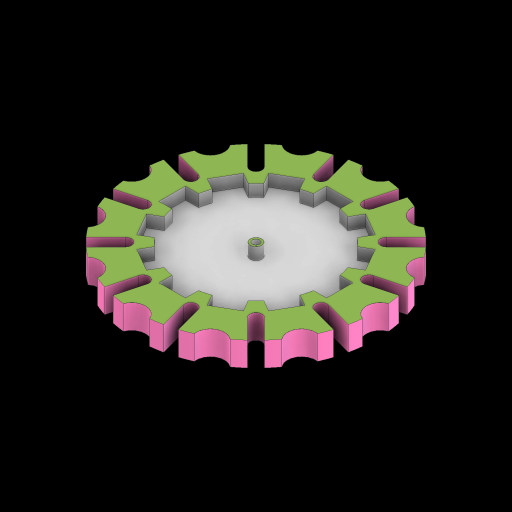
# Autodesk Inventor part: SC-1-02-Geneva Gear 12
Saved by Autodesk Inventor 2023 (Build 270158000, 158)
## iProperties
Created: 2022-10-22
Part Number: SC-1-02-Geneva Gear 12
Material: Generic
Document SubType Name: Modeling
Designer: annah
Density: 1 g/cm^3
Appearance: Default
Author: annah
Autodesk Inventor part; units mm, degrees
ref_plane "YZ Plane" through (0, 0, 0) normal (1, 0, 0) x (0, 1, 0)
ref_plane "XZ Plane" through (0, 0, 0) normal (0, 1, 0) x (-1, 0, 0)
ref_plane "XY Plane" through (0, 0, 0) normal (0, 0, 1) x (1, 0, 0)
sketch "Sketch1" plane through (0, 0, 0) normal (0, 1, 0) x (-1, 0, 0)
  line L0 (19.1342, -46.194) -> (0, -54.1231)
  line L1 (0, -54.1231) -> (0, 0)
  line L2 (0, 0) -> (19.1342, -46.194)
  circle A0 centre (0, 0) radius 50
  line L3 (17.2491, -28.6141) -> (23.8838, -44.6316)
  circle A1 centre (0, -54.1231) radius 20.712
  arc A2 (17.5355, -29.3054) -> (8.1665, -32.7812) centre (12.7859, -30.8678) ccw
  line L4 (14.5151, -48.1081) -> (8.1665, -32.7812)
  line L5 (19.1342, -41.194) -> (0, -41.194)
  circle A3 centre (0, -54.1231) radius 12.9291
  arc A4 (-11.6961, -48.6128) -> (11.6961, -48.6128) centre (0, 0) ccw
  arc A5 (-11.6961, -48.6128) -> (11.6961, -48.6128) centre (0, -54.1231) ccw
  circle A6 centre (0, -54.1231) radius 32.5
  arc A7 (19.1342, -41.194) -> (16.6765, -41.8397) centre (19.1342, -46.194) ccw
  arc A8 (14.4249, -47.874) -> (23.5974, -43.9403) centre (19.1342, -46.194) ccw
  line L6 (32.4302, -8.0362) -> (48.4477, -14.6709)
  arc A9 (33.1215, -8.3226) -> (28.9544, -17.4053) centre (30.8678, -12.7859) ccw
  line L7 (44.2813, -23.7539) -> (28.9544, -17.4053)
  arc A10 (44.052, -23.6521) -> (47.7564, -14.3846) centre (46.194, -19.1342) ccw
  circle A11 centre (38.2708, -38.2708) radius 12.9291
  line L8 (28.6141, 17.2491) -> (44.6316, 23.8838)
  arc A12 (29.3054, 17.5355) -> (32.7812, 8.1665) centre (30.8678, 12.7859) ccw
  line L9 (48.1081, 14.5151) -> (32.7812, 8.1665)
  arc A13 (47.874, 14.4249) -> (43.9403, 23.5974) centre (46.194, 19.1342) ccw
  circle A14 centre (54.1231, 0) radius 12.9291
  line L10 (8.0362, 32.4302) -> (14.6709, 48.4477)
  arc A15 (8.3226, 33.1215) -> (17.4053, 28.9544) centre (12.7859, 30.8678) ccw
  line L11 (23.7539, 44.2813) -> (17.4053, 28.9544)
  arc A16 (23.6521, 44.052) -> (14.3846, 47.7564) centre (19.1342, 46.194) ccw
  circle A17 centre (38.2708, 38.2708) radius 12.9291
  line L12 (-17.2491, 28.6141) -> (-23.8838, 44.6316)
  arc A18 (-17.5355, 29.3054) -> (-8.1665, 32.7812) centre (-12.7859, 30.8678) ccw
  line L13 (-14.5151, 48.1081) -> (-8.1665, 32.7812)
  arc A19 (-14.4249, 47.874) -> (-23.5974, 43.9403) centre (-19.1342, 46.194) ccw
  circle A20 centre (0, 54.1231) radius 12.9291
  line L14 (-32.4302, 8.0362) -> (-48.4477, 14.6709)
  arc A21 (-33.1215, 8.3226) -> (-28.9544, 17.4053) centre (-30.8678, 12.7859) ccw
  line L15 (-44.2813, 23.7539) -> (-28.9544, 17.4053)
  arc A22 (-44.052, 23.6521) -> (-47.7564, 14.3846) centre (-46.194, 19.1342) ccw
  circle A23 centre (-38.2708, 38.2708) radius 12.9291
  line L16 (-28.6141, -17.2491) -> (-44.6316, -23.8838)
  arc A24 (-29.3054, -17.5355) -> (-32.7812, -8.1665) centre (-30.8678, -12.7859) ccw
  line L17 (-48.1081, -14.5151) -> (-32.7812, -8.1665)
  arc A25 (-47.874, -14.4249) -> (-43.9403, -23.5974) centre (-46.194, -19.1342) ccw
  circle A26 centre (-54.1231, 0) radius 12.9291
  line L18 (-8.0362, -32.4302) -> (-14.6709, -48.4477)
  arc A27 (-8.3226, -33.1215) -> (-17.4053, -28.9544) centre (-12.7859, -30.8678) ccw
  line L19 (-23.7539, -44.2813) -> (-17.4053, -28.9544)
  arc A28 (-23.6521, -44.052) -> (-14.3846, -47.7564) centre (-19.1342, -46.194) ccw
  circle A29 centre (-38.2708, -38.2708) radius 12.9291
  circle A30 centre (0, 0) radius 3.5
  circle A31 centre (0, -54.1231) radius 3.5
  arc A32 (-7.5, -54.1231) -> (7.5, -54.1231) centre (0, -54.1231) ccw
  arc A33 (7.5, 0) -> (-7.5, 0) centre (0, 0) ccw
  line L20 (7.5, 0) -> (7.5, -54.1231)
  line L21 (-7.5, 0) -> (-7.5, -54.1231)
  circle A34 centre (0, -33.4111) radius 5
  point P0 (8.1662, -32.7805)
  point P1 (23.5974, -43.9403)
  point P2 (28.9537, -17.405)
  point P3 (29.1285, -29.1285)
  point P4 (26.1041, -42.6448)
  point P5 (42.6448, -26.1041)
  point P6 (32.7805, 8.1662)
  point P7 (41.194, 0)
  point P8 (48.6128, -11.6961)
  point P9 (48.6128, 11.6961)
  point P10 (17.405, 28.9537)
  point P11 (29.1285, 29.1285)
  point P12 (42.6448, 26.1041)
  point P13 (26.1041, 42.6448)
  point P14 (-8.1662, 32.7805)
  point P15 (0, 41.194)
  point P16 (11.6961, 48.6128)
  point P17 (-11.6961, 48.6128)
  point P18 (-28.9537, 17.405)
  point P19 (-29.1285, 29.1285)
  point P20 (-26.1041, 42.6448)
  point P21 (-42.6448, 26.1041)
  point P22 (-32.7805, -8.1662)
  point P23 (-41.194, 0)
  point P24 (-48.6128, 11.6961)
  point P25 (-48.6128, -11.6961)
  point P26 (-17.405, -28.9537)
  point P27 (-29.1285, -29.1285)
  point P28 (-42.6448, -26.1041)
  point P29 (-26.1041, -42.6448)
  point P30 (23.6521, -44.052)
  point P31 (26.1041, -42.6448)
  point P32 (42.6448, -26.1041)
  point P33 (44.049, -23.6577)
  point P34 (47.874, -14.4249)
  point P35 (48.6128, -11.6961)
  point P36 (48.6128, 11.6961)
  point P37 (47.8758, 14.4189)
  point P38 (44.052, 23.6521)
  point P39 (42.6448, 26.1041)
  point P40 (26.1041, 42.6448)
  point P41 (23.6577, 44.049)
  point P42 (14.4249, 47.874)
  point P43 (11.6961, 48.6128)
  point P44 (-11.6961, 48.6128)
  point P45 (-14.4189, 47.8758)
  point P46 (-23.6521, 44.052)
  point P47 (-26.1041, 42.6448)
  point P48 (-42.6448, 26.1041)
  point P49 (-44.049, 23.6577)
  point P50 (-47.874, 14.4249)
  point P51 (-48.6128, 11.6961)
  point P52 (-48.6128, -11.6961)
  point P53 (-47.8758, -14.4189)
  point P54 (-44.052, -23.6521)
  point P55 (-42.6448, -26.1041)
  point P56 (-26.1041, -42.6448)
  point P57 (-23.6577, -44.049)
  point P58 (-14.4249, -47.874)
  point P59 (14.4189, -47.8758)
  dimension "d2" = 100
  dimension "d3" = 22.5
  dimension "d4" = 20.712
  dimension "d5" = 50
  dimension "d6" = 54.1231
  dimension "d7" = 10
  dimension "d8" = 25.8582
  dimension "d9" = 65
  dimension "d10" = 360
  dimension "d11" = 7
  dimension "d12" = 7
  dimension "d13" = 15
  dimension "d14" = 15
  dimension "d15" = 10
  constraints: 113 point on circle, 44 end point, 35 centre point, 28 point on line, 9 coincident, 3 tangent, 2 vertical, 1 concentric, 1 parallel, 1 perpendicular, 161 other
  measures "d2" diameter of A0
  measures "d3" angle of L2 L1
  measures "d4" distance of L0.start L0.end
  measures "d5" distance of L1.end L0.start
  measures "d6" distance of L0.end L1.end
  measures "d7" diameter of A2
  measures "d8" diameter of A3
  measures "d9" diameter of A6
  measures "d11" diameter of A30
  measures "d12" diameter of A31
  measures "d13" diameter of A32
  measures "d14" diameter of A33
  measures "d15" diameter of A34
sketch "Sketch2" plane through (0, 0, 0) normal (0, 1, 0) x (-1, 0, 0)
  circle A0 centre (0, 0) radius 100
  line L0 (0, 0) -> (18.5658, -69.2885)
  line L1 (0, 0) -> (0, -103.5276)
  arc A1 (24.6448, -72.6673) -> (14.9907, -75.2542) centre (0, 0) ccw
  circle A2 centre (25.8819, -96.5926) radius 5
  arc A3 (24.729, -72.9816) -> (15.0747, -75.5678) centre (19.8599, -74.1181) ccw
  line L2 (30.6777, -95.1782) -> (24.6448, -72.6673)
  line L3 (21.0523, -97.8867) -> (14.9907, -75.2542)
  circle A4 centre (0, -103.5276) radius 11.6229
  line L4 (21.0523, -97.8867) -> (25.8819, -96.5926)
  arc A5 (-25.8819, -96.5926) -> (26.7197, -101.5219) centre (0, -103.5276) ccw
  circle A6 centre (0, -103.5276) radius 40
  arc A7 (57.9067, -50.8394) -> (50.8389, -57.9063) centre (54.2582, -54.2582) ccw
  line L5 (67.1751, -74.2462) -> (50.6094, -57.6767)
  line L6 (74.1567, -67.0879) -> (57.6767, -50.6094)
  circle A8 centre (70.7107, -70.7107) radius 5
  circle A9 centre (51.7638, -89.6575) radius 11.6229
  arc A10 (75.5684, -15.0748) -> (72.9809, -24.7289) centre (74.1181, -19.8599) ccw
  line L7 (95.2985, -30.7115) -> (72.6673, -24.6448)
  line L8 (97.7655, -21.0214) -> (75.2542, -14.9907)
  circle A11 centre (96.5926, -25.8819) radius 5
  circle A12 centre (89.6575, -51.7638) radius 11.6229
  arc A13 (72.9816, 24.729) -> (75.5678, 15.0747) centre (74.1181, 19.8599) ccw
  line L9 (97.8867, 21.0523) -> (75.2542, 14.9907)
  line L10 (95.1782, 30.6777) -> (72.6673, 24.6448)
  circle A14 centre (96.5926, 25.8819) radius 5
  circle A15 centre (103.5276, 0) radius 11.6229
  arc A16 (50.8394, 57.9067) -> (57.9063, 50.8389) centre (54.2582, 54.2582) ccw
  line L11 (74.2462, 67.1751) -> (57.6767, 50.6094)
  line L12 (67.0879, 74.1567) -> (50.6094, 57.6767)
  circle A17 centre (70.7107, 70.7107) radius 5
  circle A18 centre (89.6575, 51.7638) radius 11.6229
  arc A19 (15.0748, 75.5684) -> (24.7289, 72.9809) centre (19.8599, 74.1181) ccw
  line L13 (30.7115, 95.2985) -> (24.6448, 72.6673)
  line L14 (21.0214, 97.7655) -> (14.9907, 75.2542)
  circle A20 centre (25.8819, 96.5926) radius 5
  circle A21 centre (51.7638, 89.6575) radius 11.6229
  arc A22 (-24.729, 72.9816) -> (-15.0747, 75.5678) centre (-19.8599, 74.1181) ccw
  line L15 (-21.0523, 97.8867) -> (-14.9907, 75.2542)
  line L16 (-30.6777, 95.1782) -> (-24.6448, 72.6673)
  circle A23 centre (-25.8819, 96.5926) radius 5
  circle A24 centre (0, 103.5276) radius 11.6229
  arc A25 (-57.9067, 50.8394) -> (-50.8389, 57.9063) centre (-54.2582, 54.2582) ccw
  line L17 (-67.1751, 74.2462) -> (-50.6094, 57.6767)
  line L18 (-74.1567, 67.0879) -> (-57.6767, 50.6094)
  circle A26 centre (-70.7107, 70.7107) radius 5
  circle A27 centre (-51.7638, 89.6575) radius 11.6229
  arc A28 (-75.5684, 15.0748) -> (-72.9809, 24.7289) centre (-74.1181, 19.8599) ccw
  line L19 (-95.2985, 30.7115) -> (-72.6673, 24.6448)
  line L20 (-97.7655, 21.0214) -> (-75.2542, 14.9907)
  circle A29 centre (-96.5926, 25.8819) radius 5
  circle A30 centre (-89.6575, 51.7638) radius 11.6229
  arc A31 (-72.9816, -24.729) -> (-75.5678, -15.0747) centre (-74.1181, -19.8599) ccw
  line L21 (-97.8867, -21.0523) -> (-75.2542, -14.9907)
  line L22 (-95.1782, -30.6777) -> (-72.6673, -24.6448)
  circle A32 centre (-96.5926, -25.8819) radius 5
  circle A33 centre (-103.5276, 0) radius 11.6229
  arc A34 (-50.8394, -57.9067) -> (-57.9063, -50.8389) centre (-54.2582, -54.2582) ccw
  line L23 (-74.2462, -67.1751) -> (-57.6767, -50.6094)
  line L24 (-67.0879, -74.1567) -> (-50.6094, -57.6767)
  circle A35 centre (-70.7107, -70.7107) radius 5
  circle A36 centre (-89.6575, -51.7638) radius 11.6229
  arc A37 (-15.0748, -75.5684) -> (-24.7289, -72.9809) centre (-19.8599, -74.1181) ccw
  line L25 (-30.7115, -95.2985) -> (-24.6448, -72.6673)
  line L26 (-21.0214, -97.7655) -> (-14.9907, -75.2542)
  circle A38 centre (-25.8819, -96.5926) radius 5
  circle A39 centre (-51.7638, -89.6575) radius 11.6229
  circle A40 centre (0, 0) radius 3
  circle A41 centre (0, -103.5276) radius 2.5
  point P0 (50.7227, -50.7227)
  point P1 (73.9009, -74.5607)
  point P2 (69.2885, -18.5658)
  point P3 (101.2804, -27.621)
  point P4 (69.2885, 18.5658)
  point P5 (101.5219, 26.7197)
  point P6 (50.7227, 50.7227)
  point P7 (74.5607, 73.9009)
  point P8 (18.5658, 69.2885)
  point P9 (27.621, 101.2804)
  point P10 (-18.5658, 69.2885)
  point P11 (-26.7197, 101.5219)
  point P12 (-50.7227, 50.7227)
  point P13 (-73.9009, 74.5607)
  point P14 (-69.2885, 18.5658)
  point P15 (-101.2804, 27.621)
  point P16 (-69.2885, -18.5658)
  point P17 (-101.5219, -26.7197)
  point P18 (-50.7227, -50.7227)
  point P19 (-74.5607, -73.9009)
  point P20 (-18.5658, -69.2885)
  point P21 (-27.621, -101.2804)
  point P22 (40.2917, -91.5236)
  point P23 (59.1159, -80.6555)
  point P24 (67.0867, -74.1578)
  point P25 (80.6555, -59.1159)
  point P26 (91.5236, -40.2917)
  point P27 (95.1777, -30.6791)
  point P28 (99.4077, -10.8682)
  point P29 (99.4077, 10.8682)
  point P30 (97.7659, 21.0199)
  point P31 (91.5236, 40.2917)
  point P32 (80.6555, 59.1159)
  point P33 (74.1578, 67.0867)
  point P34 (59.1159, 80.6555)
  point P35 (40.2917, 91.5236)
  point P36 (30.6791, 95.1777)
  point P37 (10.8682, 99.4077)
  point P38 (-10.8682, 99.4077)
  point P39 (-21.0199, 97.7659)
  point P40 (-40.2917, 91.5236)
  point P41 (-59.1159, 80.6555)
  point P42 (-67.0867, 74.1578)
  point P43 (-80.6555, 59.1159)
  point P44 (-91.5236, 40.2917)
  point P45 (-95.1777, 30.6791)
  point P46 (-99.4077, 10.8682)
  point P47 (-99.4077, -10.8682)
  point P48 (-97.7659, -21.0199)
  point P49 (-91.5236, -40.2917)
  point P50 (-80.6555, -59.1159)
  point P51 (-74.1578, -67.0867)
  point P52 (-59.1159, -80.6555)
  point P53 (-40.2917, -91.5236)
  point P54 (-30.6791, -95.1777)
  point P55 (-10.8682, -99.4077)
  point P56 (10.8682, -99.4077)
  point P57 (21.0199, -97.7659)
  dimension "d16" = 200
  dimension "d17" = 15
  dimension "d20" = 10
  dimension "d21" = 10
  dimension "d22" = 80
  dimension "d25" = 360
  dimension "d27" = 6
  dimension "d28" = 5
  constraints: 100 point on circle, 54 end point, 41 centre point, 25 point on line, 8 coincident, 1 vertical, 198 other
  measures "d17" angle of L1 L0
  measures "d20" diameter of A2
  measures "d21" diameter of A3
  measures "d22" diameter of A6
  measures "d27" diameter of A40
  measures "d28" diameter of A41
extrude "Extrusion1" add sketch "Sketch2" along normal blind 20 contours L26 A37 A1 L1 A4 A0 | A0 A6 A1 A37 L25 | A0 A39 L24 A34 A1 A6 | L1 A1 A3 L3 A0 A4 | A37 A6 L1 A1 | A6 A37 A1 | A1 A34 A31 A28 A25 A22 A19 A16 A13 A10 A7 A6 A3 L0 A40 L1 A37 | L1 A6 L0 A3 A1 | A6 A1 A7 L5 A0 A9 | A0 L2 A3 A1 A6 | L1 A40 L0 A6 | A34 L23 A0 A36 L22 A31 A1 | A1 A3 A6 | A6 A3 L0 | A31 L21 A0 A33 L20 A28 A1 | A1 A10 L7 A0 A12 L6 A7 | A28 L19 A0 A30 L18 A25 A1 | A1 A13 L9 A0 A15 L8 A10 | A25 L17 A0 A27 L16 A22 A1 | A1 A16 L11 A0 A18 L10 A13 | A22 L15 A0 A24 L14 A19 A1 | A1 A19 L13 A0 A21 L12 A16 picked at (-24.7526, -72.3861)
sketch "Sketch3" plane through (0, 20, 0) normal (0, 1, 0) x (1, 0, 0)
  circle A0 centre (0, 0) radius 3 projected
  line L0 (-11.0031, 74.0969) -> (11.0031, 74.0969)
  line L1 (11.0031, 74.0969) -> (11.0031, 56.269)
  line L2 (11.0031, 56.269) -> (-11.0031, 56.269)
  line L3 (-11.0031, 56.269) -> (-11.0031, 74.0969)
  line L4 (11.0031, 74.0969) -> (0, 65.183) construction
  line L5 (-27.5195, 69.6713) -> (-18.6056, 54.232)
  line L6 (-18.6056, 54.232) -> (-37.6635, 43.2289)
  line L7 (-37.6635, 43.2289) -> (-46.5774, 58.6682)
  line L8 (-46.5774, 58.6682) -> (-27.5195, 69.6713)
  line L9 (-58.6682, 46.5774) -> (-43.2289, 37.6635)
  line L10 (-43.2289, 37.6635) -> (-54.232, 18.6056)
  line L11 (-54.232, 18.6056) -> (-69.6713, 27.5195)
  line L12 (-69.6713, 27.5195) -> (-58.6682, 46.5774)
  line L13 (-74.0969, 11.0031) -> (-56.269, 11.0031)
  line L14 (-56.269, 11.0031) -> (-56.269, -11.0031)
  line L15 (-56.269, -11.0031) -> (-74.0969, -11.0031)
  line L16 (-74.0969, -11.0031) -> (-74.0969, 11.0031)
  line L17 (-69.6713, -27.5195) -> (-54.232, -18.6056)
  line L18 (-54.232, -18.6056) -> (-43.2289, -37.6635)
  line L19 (-43.2289, -37.6635) -> (-58.6682, -46.5774)
  line L20 (-58.6682, -46.5774) -> (-69.6713, -27.5195)
  line L21 (-46.5774, -58.6682) -> (-37.6635, -43.2289)
  line L22 (-37.6635, -43.2289) -> (-18.6056, -54.232)
  line L23 (-18.6056, -54.232) -> (-27.5195, -69.6713)
  line L24 (-27.5195, -69.6713) -> (-46.5774, -58.6682)
  line L25 (-11.0031, -74.0969) -> (-11.0031, -56.269)
  line L26 (-11.0031, -56.269) -> (11.0031, -56.269)
  line L27 (11.0031, -56.269) -> (11.0031, -74.0969)
  line L28 (11.0031, -74.0969) -> (-11.0031, -74.0969)
  line L29 (27.5195, -69.6713) -> (18.6056, -54.232)
  line L30 (18.6056, -54.232) -> (37.6635, -43.2289)
  line L31 (37.6635, -43.2289) -> (46.5774, -58.6682)
  line L32 (46.5774, -58.6682) -> (27.5195, -69.6713)
  line L33 (58.6682, -46.5774) -> (43.2289, -37.6635)
  line L34 (43.2289, -37.6635) -> (54.232, -18.6056)
  line L35 (54.232, -18.6056) -> (69.6713, -27.5195)
  line L36 (69.6713, -27.5195) -> (58.6682, -46.5774)
  line L37 (74.0969, -11.0031) -> (56.269, -11.0031)
  line L38 (56.269, -11.0031) -> (56.269, 11.0031)
  line L39 (56.269, 11.0031) -> (74.0969, 11.0031)
  line L40 (74.0969, 11.0031) -> (74.0969, -11.0031)
  line L41 (69.6713, 27.5195) -> (54.232, 18.6056)
  line L42 (54.232, 18.6056) -> (43.2289, 37.6635)
  line L43 (43.2289, 37.6635) -> (58.6682, 46.5774)
  line L44 (58.6682, 46.5774) -> (69.6713, 27.5195)
  line L45 (46.5774, 58.6682) -> (37.6635, 43.2289)
  line L46 (37.6635, 43.2289) -> (18.6056, 54.232)
  line L47 (18.6056, 54.232) -> (27.5195, 69.6713)
  line L48 (27.5195, 69.6713) -> (46.5774, 58.6682)
  arc A1 (-11.0031, 60.9667) -> (-20.9544, 58.3003) centre (0, 0) ccw
  arc A2 (20.9544, 58.3003) -> (11.0031, 60.9667) centre (0, 0) ccw
  arc A3 (47.2972, 40.0123) -> (40.0123, 47.2972) centre (0, 0) ccw
  arc A4 (-40.0123, 47.2972) -> (-47.2972, 40.0123) centre (0, 0) ccw
  arc A5 (-58.3003, 20.9544) -> (-60.9667, 11.0031) centre (0, 0) ccw
  arc A6 (-60.9667, -11.0031) -> (-58.3003, -20.9544) centre (0, 0) ccw
  arc A7 (-47.2972, -40.0123) -> (-40.0123, -47.2972) centre (0, 0) ccw
  arc A8 (-20.9544, -58.3003) -> (-11.0031, -60.9667) centre (0, 0) ccw
  arc A9 (11.0031, -60.9667) -> (20.9544, -58.3003) centre (0, 0) ccw
  arc A10 (40.0123, -47.2972) -> (47.2972, -40.0123) centre (0, 0) ccw
  arc A11 (58.3003, -20.9544) -> (60.9667, -11.0031) centre (0, 0) ccw
  arc A12 (60.9667, 11.0031) -> (58.3003, 20.9544) centre (0, 0) ccw
  dimension "d36" = 360
  constraints: 98 end point, 24 point on circle, 24 point on line, 12 centre point, 3 coincident, 2 parallel, 1 horizontal, 1 perpendicular, 97 other
sketch "Sketch4" plane through (0, 20, 0) normal (0, 1, 0) x (1, 0, 0)
  line L0 (11.5029, -60.4669) -> (-11.5031, -60.4669)
  line L1 (-11.5031, -60.4669) -> (-11.5031, -74.5969)
  line L2 (-11.5031, -74.5969) -> (11.5029, -74.5969)
  line L3 (11.5029, -60.4669) -> (11.5029, -74.5969)
  line L4 (40.1952, -46.6144) -> (20.2715, -58.1174)
  line L5 (40.1952, -46.6144) -> (47.2602, -58.8513)
  line L6 (27.3365, -70.3543) -> (47.2602, -58.8513)
  line L7 (20.2715, -58.1174) -> (27.3365, -70.3543)
  line L8 (58.1173, -20.2716) -> (46.6143, -40.1954)
  line L9 (58.1173, -20.2716) -> (70.3542, -27.3366)
  line L10 (58.8512, -47.2604) -> (70.3542, -27.3366)
  line L11 (46.6143, -40.1954) -> (58.8512, -47.2604)
  line L12 (60.4669, 11.5029) -> (60.4669, -11.5031)
  line L13 (60.4669, 11.5029) -> (74.5969, 11.5029)
  line L14 (74.5969, -11.5031) -> (74.5969, 11.5029)
  line L15 (60.4669, -11.5031) -> (74.5969, -11.5031)
  line L16 (46.6144, 40.1952) -> (58.1174, 20.2715)
  line L17 (46.6144, 40.1952) -> (58.8513, 47.2602)
  line L18 (70.3543, 27.3365) -> (58.8513, 47.2602)
  line L19 (58.1174, 20.2715) -> (70.3543, 27.3365)
  line L20 (20.2716, 58.1173) -> (40.1954, 46.6143)
  line L21 (20.2716, 58.1173) -> (27.3366, 70.3542)
  line L22 (47.2604, 58.8512) -> (27.3366, 70.3542)
  line L23 (40.1954, 46.6143) -> (47.2604, 58.8512)
  line L24 (-11.5029, 60.4669) -> (11.5031, 60.4669)
  line L25 (-11.5029, 60.4669) -> (-11.5029, 74.5969)
  line L26 (11.5031, 74.5969) -> (-11.5029, 74.5969)
  line L27 (11.5031, 60.4669) -> (11.5031, 74.5969)
  line L28 (-40.1952, 46.6144) -> (-20.2715, 58.1174)
  line L29 (-40.1952, 46.6144) -> (-47.2602, 58.8513)
  line L30 (-27.3365, 70.3543) -> (-47.2602, 58.8513)
  line L31 (-20.2715, 58.1174) -> (-27.3365, 70.3543)
  line L32 (-58.1173, 20.2716) -> (-46.6143, 40.1954)
  line L33 (-58.1173, 20.2716) -> (-70.3542, 27.3366)
  line L34 (-58.8512, 47.2604) -> (-70.3542, 27.3366)
  line L35 (-46.6143, 40.1954) -> (-58.8512, 47.2604)
  line L36 (-60.4669, -11.5029) -> (-60.4669, 11.5031)
  line L37 (-60.4669, -11.5029) -> (-74.5969, -11.5029)
  line L38 (-74.5969, 11.5031) -> (-74.5969, -11.5029)
  line L39 (-60.4669, 11.5031) -> (-74.5969, 11.5031)
  line L40 (-46.6144, -40.1952) -> (-58.1174, -20.2715)
  line L41 (-46.6144, -40.1952) -> (-58.8513, -47.2602)
  line L42 (-70.3543, -27.3365) -> (-58.8513, -47.2602)
  line L43 (-58.1174, -20.2715) -> (-70.3543, -27.3365)
  line L44 (-20.2716, -58.1173) -> (-40.1954, -46.6143)
  line L45 (-20.2716, -58.1173) -> (-27.3366, -70.3542)
  line L46 (-47.2604, -58.8512) -> (-27.3366, -70.3542)
  line L47 (-40.1954, -46.6143) -> (-47.2604, -58.8512)
  circle A0 centre (0, 0) radius 5
  line L48 (-11.0031, 74.0969) -> (11.0031, 74.0969)
  line L49 (11.0031, 74.0969) -> (11.0031, 56.269)
  line L50 (11.0031, 56.269) -> (-11.0031, 56.269)
  line L51 (-11.0031, 56.269) -> (-11.0031, 74.0969)
  line L52 (11.0031, 74.0969) -> (0, 65.183) construction
  line L53 (-27.5195, 69.6713) -> (-18.6056, 54.232)
  line L54 (-18.6056, 54.232) -> (-37.6635, 43.2289)
  line L55 (-37.6635, 43.2289) -> (-46.5774, 58.6682)
  line L56 (-46.5774, 58.6682) -> (-27.5195, 69.6713)
  line L57 (-58.6682, 46.5774) -> (-43.2289, 37.6635)
  line L58 (-43.2289, 37.6635) -> (-54.232, 18.6056)
  line L59 (-54.232, 18.6056) -> (-69.6713, 27.5195)
  line L60 (-69.6713, 27.5195) -> (-58.6682, 46.5774)
  line L61 (-74.0969, 11.0031) -> (-56.269, 11.0031)
  line L62 (-56.269, 11.0031) -> (-56.269, -11.0031)
  line L63 (-56.269, -11.0031) -> (-74.0969, -11.0031)
  line L64 (-74.0969, -11.0031) -> (-74.0969, 11.0031)
  line L65 (-69.6713, -27.5195) -> (-54.232, -18.6056)
  line L66 (-54.232, -18.6056) -> (-43.2289, -37.6635)
  line L67 (-43.2289, -37.6635) -> (-58.6682, -46.5774)
  line L68 (-58.6682, -46.5774) -> (-69.6713, -27.5195)
  line L69 (-46.5774, -58.6682) -> (-37.6635, -43.2289)
  line L70 (-37.6635, -43.2289) -> (-18.6056, -54.232)
  line L71 (-18.6056, -54.232) -> (-27.5195, -69.6713)
  line L72 (-27.5195, -69.6713) -> (-46.5774, -58.6682)
  line L73 (-11.0031, -74.0969) -> (-11.0031, -56.269)
  line L74 (-11.0031, -56.269) -> (11.0031, -56.269)
  line L75 (11.0031, -56.269) -> (11.0031, -74.0969)
  line L76 (11.0031, -74.0969) -> (-11.0031, -74.0969)
  line L77 (27.5195, -69.6713) -> (18.6056, -54.232)
  line L78 (18.6056, -54.232) -> (37.6635, -43.2289)
  line L79 (37.6635, -43.2289) -> (46.5774, -58.6682)
  line L80 (46.5774, -58.6682) -> (27.5195, -69.6713)
  line L81 (58.6682, -46.5774) -> (43.2289, -37.6635)
  line L82 (43.2289, -37.6635) -> (54.232, -18.6056)
  line L83 (54.232, -18.6056) -> (69.6713, -27.5195)
  line L84 (69.6713, -27.5195) -> (58.6682, -46.5774)
  line L85 (74.0969, -11.0031) -> (56.269, -11.0031)
  line L86 (56.269, -11.0031) -> (56.269, 11.0031)
  line L87 (56.269, 11.0031) -> (74.0969, 11.0031)
  line L88 (74.0969, 11.0031) -> (74.0969, -11.0031)
  line L89 (69.6713, 27.5195) -> (54.232, 18.6056)
  line L90 (54.232, 18.6056) -> (43.2289, 37.6635)
  line L91 (43.2289, 37.6635) -> (58.6682, 46.5774)
  line L92 (58.6682, 46.5774) -> (69.6713, 27.5195)
  line L93 (46.5774, 58.6682) -> (37.6635, 43.2289)
  line L94 (37.6635, 43.2289) -> (18.6056, 54.232)
  line L95 (18.6056, 54.232) -> (27.5195, 69.6713)
  line L96 (27.5195, 69.6713) -> (46.5774, 58.6682)
  arc A1 (-11.0031, 60.9667) -> (-20.9544, 58.3003) centre (0, 0) ccw
  arc A2 (20.9544, 58.3003) -> (11.0031, 60.9667) centre (0, 0) ccw
  arc A3 (47.2972, 40.0123) -> (40.0123, 47.2972) centre (0, 0) ccw
  arc A4 (-40.0123, 47.2972) -> (-47.2972, 40.0123) centre (0, 0) ccw
  arc A5 (-58.3003, 20.9544) -> (-60.9667, 11.0031) centre (0, 0) ccw
  arc A6 (-60.9667, -11.0031) -> (-58.3003, -20.9544) centre (0, 0) ccw
  arc A7 (-47.2972, -40.0123) -> (-40.0123, -47.2972) centre (0, 0) ccw
  arc A8 (-20.9544, -58.3003) -> (-11.0031, -60.9667) centre (0, 0) ccw
  arc A9 (11.0031, -60.9667) -> (20.9544, -58.3003) centre (0, 0) ccw
  arc A10 (40.0123, -47.2972) -> (47.2972, -40.0123) centre (0, 0) ccw
  arc A11 (58.3003, -20.9544) -> (60.9667, -11.0031) centre (0, 0) ccw
  arc A12 (60.9667, 11.0031) -> (58.3003, 20.9544) centre (0, 0) ccw
  circle A13 centre (0, 0) radius 59.8407
  line L97 (-69.6713, -11.0031) -> (-49.8173, -11.0031)
  line L98 (-49.8173, -11.0031) -> (-49.8173, 11.0031)
  line L99 (-49.8173, 11.0031) -> (-69.6713, 11.0031)
  line L100 (-69.6713, 11.0031) -> (-69.6713, -11.0031)
  line L101 (-74.0969, 11.0031) -> (-56.269, 11.0031)
  line L102 (-65.8387, -25.3067) -> (-54.8356, -44.3646)
  line L103 (-48.6446, -15.3797) -> (-65.8387, -25.3067)
  line L104 (-37.6415, -34.4376) -> (-48.6446, -15.3797)
  line L105 (-54.8356, -44.3646) -> (-37.6415, -34.4376)
  line L106 (-69.6713, -27.5195) -> (-54.232, -18.6056)
  line L107 (-44.3646, -54.8356) -> (-25.3067, -65.8387)
  line L108 (-34.4376, -37.6415) -> (-44.3646, -54.8356)
  line L109 (-15.3797, -48.6446) -> (-34.4376, -37.6415)
  line L110 (-25.3067, -65.8387) -> (-15.3797, -48.6446)
  line L111 (-46.5774, -58.6682) -> (-37.6635, -43.2289)
  line L112 (-11.0031, -69.6713) -> (11.0031, -69.6713)
  line L113 (-11.0031, -49.8173) -> (-11.0031, -69.6713)
  line L114 (11.0031, -49.8173) -> (-11.0031, -49.8173)
  line L115 (11.0031, -69.6713) -> (11.0031, -49.8173)
  line L116 (-11.0031, -74.0969) -> (-11.0031, -56.269)
  line L117 (25.3067, -65.8387) -> (44.3646, -54.8356)
  line L118 (15.3797, -48.6446) -> (25.3067, -65.8387)
  line L119 (34.4376, -37.6415) -> (15.3797, -48.6446)
  line L120 (44.3646, -54.8356) -> (34.4376, -37.6415)
  line L121 (27.5195, -69.6713) -> (18.6056, -54.232)
  line L122 (54.8356, -44.3646) -> (65.8387, -25.3067)
  line L123 (37.6415, -34.4376) -> (54.8356, -44.3646)
  line L124 (48.6446, -15.3797) -> (37.6415, -34.4376)
  line L125 (65.8387, -25.3067) -> (48.6446, -15.3797)
  line L126 (58.6682, -46.5774) -> (43.2289, -37.6635)
  line L127 (69.6713, -11.0031) -> (69.6713, 11.0031)
  line L128 (49.8173, -11.0031) -> (69.6713, -11.0031)
  line L129 (49.8173, 11.0031) -> (49.8173, -11.0031)
  line L130 (69.6713, 11.0031) -> (49.8173, 11.0031)
  line L131 (74.0969, -11.0031) -> (56.269, -11.0031)
  line L132 (65.8387, 25.3067) -> (54.8356, 44.3646)
  line L133 (48.6446, 15.3797) -> (65.8387, 25.3067)
  line L134 (37.6415, 34.4376) -> (48.6446, 15.3797)
  line L135 (54.8356, 44.3646) -> (37.6415, 34.4376)
  line L136 (69.6713, 27.5195) -> (54.232, 18.6056)
  line L137 (44.3646, 54.8356) -> (25.3067, 65.8387)
  line L138 (34.4376, 37.6415) -> (44.3646, 54.8356)
  line L139 (15.3797, 48.6446) -> (34.4376, 37.6415)
  line L140 (25.3067, 65.8387) -> (15.3797, 48.6446)
  line L141 (46.5774, 58.6682) -> (37.6635, 43.2289)
  line L142 (11.0031, 69.6713) -> (-11.0031, 69.6713)
  line L143 (11.0031, 49.8173) -> (11.0031, 69.6713)
  line L144 (-11.0031, 49.8173) -> (11.0031, 49.8173)
  line L145 (-11.0031, 69.6713) -> (-11.0031, 49.8173)
  line L146 (11.0031, 74.0969) -> (11.0031, 56.269)
  line L147 (-25.3067, 65.8387) -> (-44.3646, 54.8356)
  line L148 (-15.3797, 48.6446) -> (-25.3067, 65.8387)
  line L149 (-34.4376, 37.6415) -> (-15.3797, 48.6446)
  line L150 (-44.3646, 54.8356) -> (-34.4376, 37.6415)
  line L151 (-27.5195, 69.6713) -> (-18.6056, 54.232)
  line L152 (-54.8356, 44.3646) -> (-65.8387, 25.3067)
  line L153 (-37.6415, 34.4376) -> (-54.8356, 44.3646)
  line L154 (-48.6446, 15.3797) -> (-37.6415, 34.4376)
  line L155 (-65.8387, 25.3067) -> (-48.6446, 15.3797)
  point P0 (-58.6905, -20.6023)
  point P1 (-47.1875, -40.5261)
  point P2 (-40.5263, -47.1874)
  point P3 (-20.6025, -58.6904)
  point P4 (-11.5031, -61.1286)
  point P5 (11.5029, -61.1286)
  point P6 (20.6023, -58.6905)
  point P7 (40.5261, -47.1875)
  point P8 (47.1874, -40.5263)
  point P9 (58.6904, -20.6025)
  point P10 (61.1286, -11.5031)
  point P11 (61.1286, 11.5029)
  point P12 (58.6905, 20.6023)
  point P13 (47.1875, 40.5261)
  point P14 (40.5263, 47.1874)
  point P15 (20.6025, 58.6904)
  point P16 (11.5031, 61.1286)
  point P17 (-11.5029, 61.1286)
  point P18 (-20.6023, 58.6905)
  point P19 (-40.5261, 47.1875)
  point P20 (-47.1874, 40.5263)
  point P21 (-58.6904, 20.6025)
  point P22 (-61.1286, 11.5031)
  point P23 (-61.1286, -11.5029)
  point P24 (-58.3003, -20.9544)
  point P25 (-11.0031, -60.9667)
  point P26 (20.9544, -58.3003)
  point P27 (47.2972, -40.0123)
  point P28 (60.9667, -11.0031)
  point P29 (58.3003, 20.9544)
  point P30 (40.0123, 47.2972)
  point P31 (11.0031, 60.9667)
  point P32 (-20.9544, 58.3003)
  point P33 (-45.4384, -38.9392)
  point P34 (-38.9392, -45.4384)
  point P35 (-19.8812, -56.4415)
  point P36 (-11.0031, -58.8204)
  point P37 (11.0031, -58.8204)
  point P38 (19.8812, -56.4415)
  point P39 (38.9392, -45.4384)
  point P40 (45.4384, -38.9392)
  point P41 (56.4415, -19.8812)
  point P42 (58.8204, -11.0031)
  point P43 (58.8204, 11.0031)
  point P44 (56.4415, 19.8812)
  point P45 (45.4384, 38.9392)
  point P46 (38.9392, 45.4384)
  point P47 (19.8812, 56.4415)
  point P48 (11.0031, 58.8204)
  point P49 (-11.0031, 58.8204)
  point P50 (-19.8812, 56.4415)
  point P51 (-38.9392, 45.4384)
  point P52 (-45.4384, 38.9392)
  point P53 (-56.4415, 19.8812)
  point P54 (-58.8204, 11.0031)
  point P55 (-58.8204, -11.0031)
  point P56 (-56.4415, -19.8812)
  dimension "d48" = 360
  dimension "d55" = 360
  dimension "d56" = 360
  constraints: 312 end point, 60 point on line, 24 point on circle, 13 centre point, 4 coincident, 4 parallel, 3 horizontal, 2 perpendicular, 1 vertical, 341 other
extrude "Extrusion4" cut sketch "Sketch4" against normal blind 10 contours L75 L112 L73 L0 | L0 L73 A13 L75 | A13 L73 L74 L75 | L75 L115 L114 L113 L73 A13 L71 L110 L109 L108 L69 L67 L105 L104 L103 L65 L63 L97 L98 L99 L61 L59 L155 L154 L153 L57 L55 L150 L149 L148 L53 L51 L145 L144 L143 L49 L95 L140 L139 L138 L93 L91 L135 L134 L133 L89 L87 L130 L129 L128 L85 L83 L125 L124 L123 L81 L79 L120 L119 L118 L77 | L74 L113 L114 L115 | A13 L79 L4 L77 | L77 L78 L79 A13 | L77 L4 L79 L117 | A13 L69 L70 L71 | L71 L44 L69 A13 | L118 L119 L120 L78 | L70 L108 L109 L110 | L71 L107 L69 L44 | A13 L83 L8 L81 | L81 L82 L83 A13 | A13 L65 L66 L67 | L67 L40 L65 A13 | L8 L83 L122 L81 | L123 L124 L125 L82 | L66 L103 L104 L105 | L67 L102 L65 L40 | A13 L87 L12 L85 | L85 L86 L87 A13 | A13 L61 L62 L63 | L63 L36 L61 A13 | L12 L87 L127 L85 | L128 L129 L130 L86 | L62 L99 L98 L97 | L63 L100 L61 L36 | A13 L57 L58 L59 | L59 L32 L57 A13 | A13 L91 L16 L89 | L89 L90 L91 A13 | L58 L153 L154 L155 | L59 L152 L57 L32 | L16 L91 L132 L89 | L133 L134 L135 L90 | A13 L53 L54 L55 | L55 L28 L53 A13 | A13 L95 L20 L93 | L93 L94 L95 A13 | L54 L148 L149 L150 | L55 L147 L53 L28 | L20 L95 L137 L93 | L138 L139 L140 L94 | A13 L49 L50 L51 | L51 L24 L49 A13 | L50 L143 L144 L145 | L51 L142 L49 L24
sketch "Sketch5" plane through (0, 20, 0) normal (0, 1, 0) x (1, 0, 0)
  circle A0 centre (0, 0) radius 5
  circle A1 centre (0, 0) radius 5 projected
  circle A2 centre (0, 0) radius 4.75
  dimension "d59" = 10
  dimension "d60" = 9.5
  constraints: 2 centre point, 2 coincident
  measures "d59" diameter of A0
  measures "d60" diameter of A2
extrude "Extrusion5" cut sketch "Sketch5" against normal blind 10
body "Solid1"
